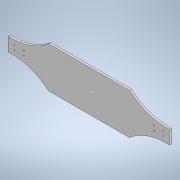
# Autodesk Inventor part: Electric Skateboard Deck
Saved by Autodesk Inventor 2020 (Build 240168000, 168)
## iProperties
Created: 2019-09-21
Part Number: Electric Skateboard Deck
Material: Generic
Document SubType Name: Modeling
Designer: User
Density: 1 g/cm^3
Appearance: Default
Author: User
Autodesk Inventor part; units mm, degrees
ref_plane "YZ Plane" through (0, 0, 0) normal (1, 0, 0) x (0, 1, 0)
ref_plane "XZ Plane" through (0, 0, 0) normal (0, 1, 0) x (-1, 0, 0)
ref_plane "XY Plane" through (0, 0, 0) normal (0, 0, 1) x (1, 0, 0)
sketch "Sketch1" plane through (0, 0, 0) normal (0, 0, 1) x (1, 0, 0)
  line L0 (726.3915, 245.3629) -> (1226.3925, 245.3629)
  line L1 (1476.392, 160.6963) -> (1476.392, 76.0296)
  line L2 (476.392, 76.0296) -> (476.392, 160.6963)
  arc A0 (476.392, 160.6963) -> (726.3915, 245.3629) centre (495.472, 515.784) ccw
  line L3 (1476.392, 118.3629) -> (476.392, 118.3629) construction
  line L4 (976.392, -8.6371) -> (976.392, 245.3629) construction
  arc A1 (726.3915, -8.6371) -> (476.392, 76.0296) centre (495.472, -279.0582) ccw
  arc A2 (1226.3925, 245.3629) -> (1476.392, 160.6963) centre (1457.312, 515.784) ccw
  arc A3 (1476.392, 76.0296) -> (1226.3925, -8.6371) centre (1457.312, -279.0582) ccw
  line L5 (726.3915, -8.6371) -> (1226.3925, -8.6371)
  point P0 (0, 0)
  dimension "d4" = 355.6
  dimension "d5" = 254
  dimension "d6" = 84.6667
  constraints: 12 end point, 9 symmetric about line, 8 point on circle, 4 centre point, 3 midpoint, 2 horizontal, 2 perpendicular, 1 parallel, 1 vertical, 3 other
  measures "d4" radius of A0
  measures "d5" distance of L5.end L0.end
  measures "d6" distance of L1.end L1.start
extrude "Extrusion1" add sketch "Sketch1" along normal blind 12.7
sketch "Sketch2" plane through (0, 0, 12.7) normal (0, 0, 1) x (1, 0, 0)
  point P0 (0, 0)
move or copy body "Move Body1" bodies to move or copy 1 copy no translate (-1000.125, -123.825, 0)
sketch "Sketch3" plane through (-273.7335, 121.5379, 12.7) normal (0, 0, 1) x (1, 0, 0)
  line L0 (-249.9995, -84.6667) -> (-249.9995, -169.3333) construction
  arc A0 (750.0005, -169.3333) -> (500.001, -254) centre (730.9205, -524.4211) ccw projected
  line L1 (-249.9995, -84.6667) -> (750.0005, -84.6667) construction
  line L2 (750.0005, -84.6667) -> (750.0005, -169.3333) construction
  line L3 (750.0005, -169.3333) -> (-249.9995, -169.3333) construction
  line L4 (-249.9995, -169.3333) -> (-249.9995, -84.6667) construction
  line L5 (-249.9995, -84.6667) -> (-249.9995, -112.8861) construction
  line L6 (750.0005, -169.3333) -> (750.0005, -84.6667) construction
  line L7 (-249.9995, -112.8861) -> (750.0005, -112.8861) construction
  line L8 (750.0005, -112.8861) -> (750.0005, -141.1055) construction
  line L9 (750.0005, -141.1055) -> (-249.9995, -141.1055) construction
  line L10 (-249.9995, -141.1055) -> (-249.9995, -112.8861) construction
  arc A1 (-249.9995, -84.6667) -> (0, 0) centre (-230.9195, 270.4211) ccw projected
  line L11 (-211.8394, -84.6667) -> (-211.8394, -169.3333) construction
  arc A2 (0, -254) -> (-249.9995, -169.3333) centre (-230.9195, -524.4211) ccw projected
  line L12 (-211.8394, -84.6667) -> (-153.2669, -84.6667) construction
  line L13 (-153.2669, -84.6667) -> (-153.2669, -169.3333) construction
  line L14 (-153.2669, -169.3333) -> (-211.8394, -169.3333) construction
  line L15 (-211.8394, -169.3333) -> (-211.8394, -84.6667) construction
  line L16 (500.001, 0) -> (0, 0) projected
  line L17 (250.0005, 0) -> (250.0005, -254) construction
  point P0 (273.7335, -121.5379)
  point P1 (-211.8394, -112.8861)
  point P2 (-211.8394, -141.1055)
  point P3 (-153.2669, -112.8861)
  point P4 (-153.2669, -141.1055)
  point P5 (711.8404, -112.8861)
  point P6 (711.8404, -141.1055)
  point P7 (653.2679, -112.8861)
  point P8 (653.2679, -141.1055)
  dimension "d15" = 28.2194
  dimension "d16" = 28.2194
  constraints: 30 end point, 13 point on line, 6 parallel, 4 symmetric about line, 3 horizontal, 3 perpendicular, 2 point on circle, 1 midpoint, 1 vertical
  measures "d15" distance of L0.start L5.end
  measures "d16" distance of L7.end L8.end
hole "Hole1" at (-485.5729, 8.6519, 12.7) at (-427.0004, 8.6519, 12.7) at (-485.5729, -19.5675, 12.7) at (-427.0004, -19.5675, 12.7) at (379.5345, 8.6519, 12.7) at (438.1069, 8.6519, 12.7) at (438.1069, -19.5675, 12.7) at (379.5345, -19.5675, 12.7) direction (0, 0, -1) diameter 6.35 end through all
thread "Thread1" size "1/4-20 UNC" class "2B" standard "ANSI Unified Screw Threads" full length
body "Solid1"
